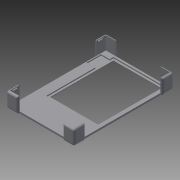
# Autodesk Inventor part: TouchBottom
Saved by Autodesk Inventor 2014 SP1 (Build 180222100, 222)
## iProperties
Created: 2014-03-24
Part Number: TouchBottom
Material: Generic
Document SubType Name: Modeling
Designer: patrigg
Density: 1 g/cm^3
Appearance: Default
Author: patrigg
Autodesk Inventor part; units mm, degrees
ref_plane "YZ Plane" through (0, 0, 0) normal (1, 0, 0) x (0, 1, 0)
ref_plane "XZ Plane" through (0, 0, 0) normal (0, 1, 0) x (-1, 0, 0)
ref_plane "XY Plane" through (0, 0, 0) normal (0, 0, 1) x (1, 0, 0)
sketch "Sketch1" plane through (0, 0, 0) normal (0, 1, 0) x (-1, 0, 0)
  line L0 (-33.5, -50) -> (33.5, -50)
  line L1 (33.5, -50) -> (33.5, 50)
  line L2 (33.5, 50) -> (-33.5, 50)
  line L3 (-33.5, 50) -> (-33.5, -50)
  line L4 (-33.5, -50) -> (33.5, 50) construction
  line L5 (33.5, -50) -> (-33.5, 50) construction
  point P0 (0, 0)
  dimension "d0" = 67
  dimension "d1" = 100
  constraints: 12 end point, 2 midpoint, 2 parallel, 1 horizontal, 1 perpendicular
  measures "d0" distance of L2.end L1.end
  measures "d1" distance of L1.end L0.end
extrude "Extrusion1" add sketch "Sketch1" along normal blind 1.8
sketch "Sketch2" plane through (0, 1.8, 0) normal (0, 1, 0) x (1, 0, 0)
  line L0 (33.5, 50) -> (-33.5, 50) projected
  line L1 (-23.5, -22) -> (32.5, -22)
  line L2 (32.5, -22) -> (32.5, 48)
  line L3 (32.5, 48) -> (-23.5, 48)
  line L4 (-23.5, 48) -> (-23.5, -22)
  line L5 (-23.5, -22) -> (32.5, 48) construction
  line L6 (32.5, -22) -> (-23.5, 48) construction
  line L7 (33.5, -50) -> (33.5, 50) projected
  point P0 (0, 0)
  point P1 (4.5, 13)
  point P2 (4.5, 13)
  dimension "d5" = 56
  dimension "d6" = 70
  dimension "d7" = 2
  dimension "d33" = 1
  constraints: 12 end point, 3 midpoint, 2 parallel, 1 horizontal, 1 perpendicular
  measures "d5" distance of L3.end L2.end
  measures "d6" distance of L2.end L1.end
  measures "d7" distance between parallel lines of L0 L3
  measures "d33" distance between parallel lines of L7 L2
extrude "Extrusion2" cut sketch "Sketch2" against normal blind 1.1
sketch "Sketch3" plane through (0, 0.7, 0) normal (0, 1, 0) x (1, 0, 0)
  line L0 (32.5, -22) -> (-23.5, -22) projected
  line L1 (32.5, 48) -> (32.5, -22) projected
  line L2 (-23.5, 48) -> (32.5, 48) projected
  line L3 (-23.5, -22) -> (-23.5, 48) projected
  line L4 (-21.5, 46) -> (28.5, 46)
  line L5 (28.5, 46) -> (28.5, -20)
  line L6 (28.5, -20) -> (-21.5, -20)
  line L7 (-21.5, -20) -> (-21.5, 46)
  point P0 (0, 0)
  dimension "d10" = 2
  dimension "d11" = 2
  dimension "d12" = 4
  dimension "d13" = 2
  constraints: 8 end point, 2 parallel, 1 horizontal, 1 perpendicular
  measures "d10" distance between parallel lines of L2 L4
  measures "d11" distance between parallel lines of L3 L7
  measures "d12" distance between parallel lines of L1 L5
  measures "d13" distance between parallel lines of L0 L6
extrude "Extrusion3" cut sketch "Sketch3" against normal blind 1 contours L4 L5 L6 L7
sketch "Sketch7" plane through (0, 1.8, 0) normal (0, 1, 0) x (1, 0, 0)
  line L0 (-23.5, -22) -> (-23.5, 48) projected
  line L1 (33.5, 50) -> (-33.5, 50) projected
  line L2 (-33.5, 50) -> (-33.5, -50) projected
  line L3 (-23.5, 44) -> (-32.5, 44)
  line L4 (-32.5, 44) -> (-32.5, 29)
  line L5 (-32.5, 29) -> (-23.5, 29)
  line L6 (-23.5, 29) -> (-23.5, 44)
  point P0 (0, 0)
  dimension "d28" = 1
  dimension "d29" = 6
  dimension "d30" = 15
  constraints: 8 end point, 2 parallel, 1 horizontal, 1 perpendicular, 1 point on line
  measures "d28" distance between parallel lines of L4 L2
  measures "d29" distance between parallel lines of L3 L1
  measures "d30" distance between parallel lines of L5 L3
extrude "Extrusion6" cut sketch "Sketch7" against normal up to surface (1.1 mm away)
sketch "Sketch9" plane through (0, 0, 0) normal (0, -1, 0) x (1, 0, 0)
  line L0 (33.5, -50) -> (-33.5, -50) projected
  line L1 (33.5, 50) -> (33.5, -50) projected
  line L2 (-33.5, 50) -> (33.5, 50) projected
  line L3 (-33.5, -50) -> (-33.5, 50) projected
  line L4 (-33.5, 40) -> (-35.5, 40)
  line L5 (-35.5, 40) -> (-35.5, 52)
  line L6 (-35.5, 52) -> (-23.5, 52)
  line L7 (-23.5, 52) -> (-23.5, 50)
  line L8 (23.5, 50) -> (23.5, 52)
  line L9 (23.5, 52) -> (35.5, 52)
  line L10 (35.5, 52) -> (35.5, 40)
  line L11 (35.5, 40) -> (33.5, 40)
  line L12 (33.5, -40) -> (35.5, -40)
  line L13 (35.5, -40) -> (35.5, -52)
  line L14 (35.5, -52) -> (23.5, -52)
  line L15 (23.5, -52) -> (23.5, -50)
  line L16 (-23.5, -50) -> (-23.5, -52)
  line L17 (-23.5, -52) -> (-35.5, -52)
  line L18 (-35.5, -52) -> (-35.5, -40)
  line L19 (-35.5, -40) -> (-33.5, -40)
  point P0 (0, 0)
  dimension "d34" = 2
  dimension "d35" = 2
  dimension "d36" = 2
  dimension "d37" = 2
  dimension "d38" = 10
  dimension "d39" = 10
  dimension "d40" = 10
  dimension "d41" = 10
  constraints: 32 end point, 9 parallel, 8 collinear, 8 point on line, 7 perpendicular
  measures "d34" distance between parallel lines of L2 L6
  measures "d35" distance between parallel lines of L3 L5
  measures "d36" distance between parallel lines of L0 L14
  measures "d37" distance between parallel lines of L1 L13
  measures "d38" distance of L7.end L2.start
  measures "d39" distance of L4.start L2.start
  measures "d40" distance of L0.start L12.start
  measures "d41" distance of L0.start L15.end
extrude "Extrusion7" add sketch "Sketch9" against normal blind 15.6 contours L1 L12 L13 L14 L15 L0 | L16 L17 L18 L19 L3 L0 | L1 L2 L8 L9 L10 L11 | L4 L5 L6 L7 L2 L3
fillet "Fillet1" radius 2 28 edges at (-29.5, 15.6, 52) (-35.5, 15.6, 46) (-35.5, 7.8, 52) (-23.5, 7.8, 52) (-29.5, 0, 52) (29.5, 0, 52) (23.5, 7.8, 52) (29.5, 15.6, 52) (35.5, 7.8, 52) (35.5, 15.6, 46) (35.5, 7.8, 40) (35.5, 0, 46) (35.5, 7.8, -40) (35.5, 15.6, -46) (35.5, 7.8, -52) (35.5, 0, -46) (29.5, 0, -52) (23.5, 7.8, -52) (29.5, 15.6, -52) (-35.5, 7.8, -40) (-35.5, 15.6, -46) (-35.5, 7.8, -52) (-29.5, 15.6, -52) (-23.5, 7.8, -52) (-29.5, 0, -52) (-35.5, 0, -46) (-35.5, 0, 46) (-35.5, 7.8, 40)
sketch "Sketch10" plane through (-33.5, 1.8, -50) normal (1, 0, 0) x (0, 0, -1)
  line L0 (0, 0) -> (0, 13.8) projected
  line L1 (-10, 13.8) -> (0, 13.8) projected
  line L2 (-10, 0) -> (-10, 13.8) projected
  line L3 (-10, 12) -> (0, 12) construction
  line L4 (-8, 13) -> (-3, 13)
  line L5 (-3, 13) -> (-3, 12)
  line L6 (-3, 12) -> (-8, 12)
  line L7 (-8, 12) -> (-8, 13)
  point P0 (-50, -1.8)
  dimension "d45" = 1.8
  dimension "d46" = 1
  dimension "d47" = 2
  dimension "d48" = 5
  constraints: 10 end point, 3 point on line, 2 parallel, 2 perpendicular, 1 horizontal
  measures "d45" distance between parallel lines of L3 L1
  measures "d46" distance between parallel lines of L3 L4
  measures "d47" distance between parallel lines of L2 L7
  measures "d48" distance between parallel lines of L7 L5
extrude "Extrusion9" cut sketch "Sketch10" against normal blind 1 draft -10
sketch "Sketch12" plane through (-33.5, 1.8, 40) normal (1, 0, 0) x (0, 0, -1)
  line L0 (0, 0) -> (0, 13.8) projected
  line L1 (-7, 12.8237) -> (-2, 12.8237)
  line L2 (-2, 12.8237) -> (-2, 11.8237)
  line L3 (-2, 11.8237) -> (-7, 11.8237)
  line L4 (-7, 11.8237) -> (-7, 12.8237)
  line L5 (86.8237, 12.8237) -> (82.1763, 12.8237) projected
  point P0 (40, -1.8)
  dimension "d56" = 5
  dimension "d57" = 1
  dimension "d59" = 2
  constraints: 8 end point, 2 parallel, 1 collinear, 1 horizontal, 1 perpendicular
  measures "d56" distance of L2.end L3.end
  measures "d57" distance of L1.end L2.end
  measures "d59" distance from line of L0 L1.end
extrude "Extrusion10" cut sketch "Sketch12" against normal blind 1 draft -10
sketch "Sketch13" plane through (33.5, 1.8, 50) normal (-1, 0, 0) x (0, 0, 1)
  line L0 (-8, 11.8237) -> (-3, 11.8237) projected
  line L1 (-3, 11.8237) -> (-3, 12.8237) projected
  line L2 (-3, 12.8237) -> (-8, 12.8237) projected
  line L3 (-8, 12.8237) -> (-8, 11.8237) projected
  line L4 (-8, 12.8237) -> (-3, 12.8237)
  line L5 (-3, 12.8237) -> (-3, 11.8237)
  line L6 (-3, 11.8237) -> (-8, 11.8237)
  line L7 (-8, 11.8237) -> (-8, 12.8237)
  point P0 (-50, -1.8)
  constraints: 8 end point, 2 parallel, 1 horizontal, 1 perpendicular
extrude "Extrusion11" cut sketch "Sketch13" against normal blind 1 draft -10
sketch "Sketch14" plane through (33.5, 1.8, -40) normal (-1, 0, 0) x (0, 0, 1)
  line L0 (-7, 12) -> (-2, 12) projected
  line L1 (-7, 13) -> (-7, 12) projected
  line L2 (-2, 12) -> (-2, 13) projected
  line L3 (-2, 13) -> (-7, 13) projected
  point P0 (40, -1.8)
extrude "Extrusion12" cut sketch "Sketch14" against normal blind 1 draft -10
body "Solid1"
